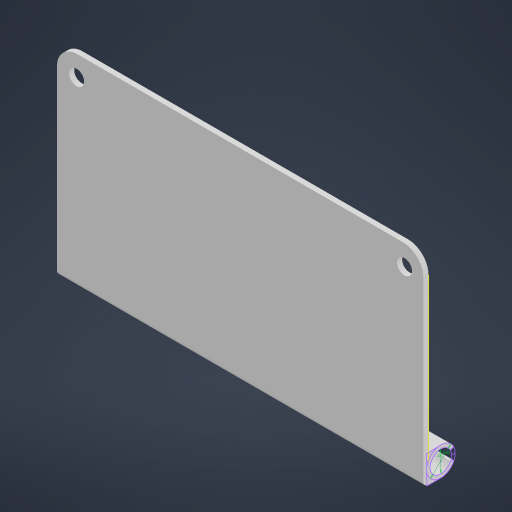
# Autodesk Inventor part: plate holder holder
Saved by Autodesk Inventor 2024 (Build 280153000, 153)
## iProperties
Created: 2023-07-26
Part Number: plate holder holder
Material: Generic
Document SubType Name: Modeling
Designer: reima
Density: 1 g/cm^3
Appearance: Default
Author: reima
Autodesk Inventor part; units mm, degrees
ref_plane "YZ Plane" through (0, 0, 0) normal (1, 0, 0) x (0, 1, 0)
ref_plane "XZ Plane" through (0, 0, 0) normal (0, 1, 0) x (-1, 0, 0)
ref_plane "XY Plane" through (0, 0, 0) normal (0, 0, 1) x (1, 0, 0)
sketch "Sketch1" plane through (0, 0, 0) normal (1, 0, 0) x (0, 1, 0)
  point P0 (0, 0)
sketch "Sketch2" plane through (0, 0, 0) normal (0, 0, 1) x (1, 0, 0)
  circle A0 centre (13.979, 17.0432) radius 2.3368 projected
  circle A1 centre (13.725, -33.7568) radius 2.3368 projected
  circle A2 centre (-87.875, -33.7568) radius 2.3368 projected
  circle A3 centre (-87.875, 17.0432) radius 2.3368 projected
  line L0 (-87.621, -39.5988) -> (13.471, -39.5988) projected
  arc A4 (-93.971, -33.2488) -> (-87.621, -39.5988) centre (-87.621, -33.2488) ccw projected
  line L1 (-93.971, 17.0432) -> (-93.971, -33.2488) projected
  arc A5 (-87.621, 23.3932) -> (-93.971, 17.0432) centre (-87.621, 17.0432) ccw projected
  line L2 (13.471, 23.3932) -> (-87.621, 23.3932) projected
  arc A6 (19.821, 17.0432) -> (13.471, 23.3932) centre (13.471, 17.0432) ccw projected
  line L3 (19.821, -33.2488) -> (19.821, 17.0432) projected
  arc A7 (13.471, -39.5988) -> (19.821, -33.2488) centre (13.471, -33.2488) ccw projected
  circle A8 centre (13.725, -33.7568) radius 2.3368 projected
  circle A9 centre (13.979, 17.0432) radius 2.3368 projected
  circle A10 centre (-87.875, -33.7568) radius 2.3368 projected
  circle A11 centre (-87.875, 17.0432) radius 2.3368 projected
  point P0 (0, 0)
extrude "Extrusion1" add sketch "Sketch2" along normal blind 1.5875
sketch "Sketch3" plane through (19.821, -33.2488, 0) normal (1, 0, 0) x (0, 0, -1)
  circle A0 centre (3.7949, -1.7964) radius 3.3655
  circle A1 centre (3.7949, -1.7964) radius 4.445
  line L0 (3.1599, 2.6031) -> (-0.6501, 2.4684)
  line L1 (-0.6501, 2.4684) -> (-0.6501, -1.7964)
  line L2 (-0.6501, -1.7964) -> (-0.493, -6.2414)
  line L3 (-0.493, -6.2414) -> (3.7949, -6.2414)
  line L4 (0, 0) -> (0, 50.292) projected
  line L5 (7.1604, -1.7964) -> (8.2399, -1.7964)
  line L6 (6.8216, -0.3249) -> (7.744, 0.2439)
  line L7 (6.8216, -3.2678) -> (7.8694, -3.5728)
  point P0 (0, 33.2488)
  point P1 (0, 2.4914)
  point P2 (0, 1.3549)
  point P3 (-0.6391, -2.1102)
  point P4 (0, 0.5182)
  dimension "d2" = 6.731
  dimension "d3" = 8.89
  constraints: 14 end point, 9 point on circle, 2 centre point, 2 tangent, 1 coincident, 1 horizontal, 1 perpendicular
  measures "d2" diameter of A0
  measures "d3" diameter of A1
extrude "Extrusion2" add sketch "Sketch3" against normal up to surface (113.792 mm away) contours L5 A1 L7 A0 | A0 L6 A1 L5 | A0 L7 A1 L6 | A1 L4 L0
sketch "Sketch4" plane through (0, 0, 1.5875) normal (0, 0, 1) x (1, 0, 0)
  circle A0 centre (13.725, -33.7568) radius 2.3368 projected
  line L0 (19.821, -39.4902) -> (-93.971, -39.4902) projected
  line L1 (19.821, -39.4902) -> (19.821, -30.6002) projected
  line L2 (19.821, -30.7575) -> (-93.971, -30.7575) projected
  line L3 (19.821, -39.4902) -> (-93.971, -39.4902)
  line L4 (-93.971, -39.4902) -> (-93.971, -30.7575)
  line L5 (-93.971, -30.7575) -> (19.821, -30.7575)
  line L6 (19.821, -30.7575) -> (19.821, -39.4902)
  circle A1 centre (-87.875, -33.7568) radius 2.3368 projected
  circle A2 centre (-87.875, 17.0432) radius 2.3368 projected
  circle A3 centre (-87.875, 17.0432) radius 2.921
  circle A4 centre (13.979, 17.0432) radius 2.3368 projected
  circle A5 centre (13.979, 17.0432) radius 2.921
  point P0 (0, 0)
  point P1 (19.821, -33.2488)
  point P2 (19.821, -30.6458)
  dimension "d6" = 5.842
  dimension "d7" = 5.842
  constraints: 8 end point, 2 centre point, 2 coincident, 2 parallel, 1 horizontal, 1 perpendicular
  measures "d6" diameter of A3
  measures "d7" diameter of A5
extrude "Extrusion3" add sketch "Sketch4" against normal up to surface contours A0 | L0 L4 L2 L1 | A1
sketch "Sketch5" plane through (19.821, 17.0432, 1.5875) normal (1, 0, 0) x (0, 0, -1)
  line L0 (0, -56.5334) -> (0, -56.642) projected
  line L1 (0, -56.5334) -> (1.6302, -56.5334)
  line L2 (1.6302, -56.5334) -> (1.6302, -56.6709)
  line L3 (1.6302, -56.6709) -> (0, -56.6709)
  line L4 (0, -56.6709) -> (0, -56.5334)
  point P0 (1.5875, -17.0432)
  constraints: 8 end point, 2 parallel, 1 horizontal, 1 perpendicular
extrude "Extrusion4" cut sketch "Sketch5" against normal blind 136.017
fillet "Fillet1" radius 1.5875 1 edges at (-37.075, -39.4902, 1.5875)
sketch "Sketch6" plane through (-93.971, 17.0432, 0) normal (-1, 0, 0) x (0, 0, 1)
  circle A0 centre (-3.7949, -52.0884) radius 3.3655 projected
  line L0 (-7.1604, -52.0884) -> (-8.2399, -52.0884)
  arc A1 (-3.1599, -47.6889) -> (-3.7949, -56.5334) centre (-3.7949, -52.0884) ccw projected
  line L1 (-7.4629, -53.118) -> (-8.0595, -53.3483)
  line L2 (-7.4629, -51.0587) -> (-8.0595, -50.8284)
  point P0 (0, -17.0432)
  point P1 (-7.4631, -51.0586)
  point P2 (-8.0577, -50.8291)
  point P3 (-8.0577, -53.3476)
  point P4 (-7.4631, -53.1181)
  constraints: 6 end point, 2 symmetric about line, 1 horizontal, 1 point on circle, 2 other
extrude "Extrusion6" cut sketch "Sketch3" against normal blind 115.8875 contours L5 A1 L7 A0 | A0 L6 A1 L5
body "Solid1"
